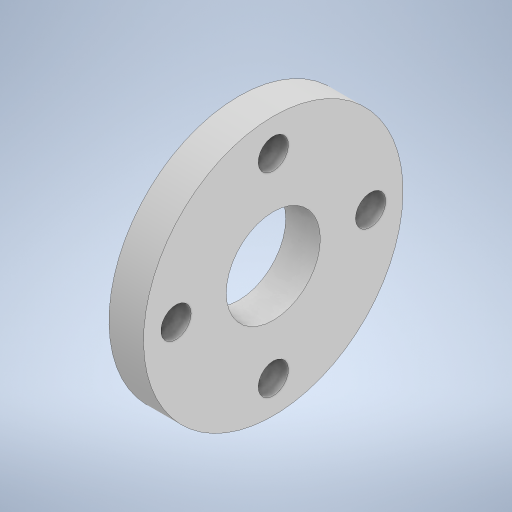
# Autodesk Inventor part: 06-01-2023 flangia piccola
Saved by Autodesk Inventor 2023 (Build 270158000, 158)
## iProperties
Created: 2023-05-31
Part Number: 06-01-2023 flangia piccola
Material: Generico
Document SubType Name: Modeling
Designer: Admin
Density: 1 g/cm^3
Appearance: Default
Author: Admin
Autodesk Inventor part; units mm, degrees
ref_plane "YZ Plane" through (0, 0, 0) normal (1, 0, 0) x (0, 1, 0)
ref_plane "XZ Plane" through (0, 0, 0) normal (0, 1, 0) x (-1, 0, 0)
ref_plane "XY Plane" through (0, 0, 0) normal (0, 0, 1) x (1, 0, 0)
sketch "Schizzo1" plane through (0, 0, 0) normal (0, 0, 1) x (1, 0, 0)
  line L0 (0, 0) -> (22.1221, 0) construction
  line L1 (0, 0) -> (0, 21.75) construction
  line L2 (0, 60) -> (16, 60)
  line L3 (16, 60) -> (16, 21.75)
  line L4 (16, 21.75) -> (0, 21.75)
  line L5 (0, 21.75) -> (0, 60)
  dimension "d0" = 16
  dimension "d1" = 38.25
  dimension "d2" = 120
  constraints: 12 end point, 3 perpendicular, 1 horizontal, 1 parallel, 1 point on line, 1 vertical
  measures "d0" distance of L2.start L2.end
  measures "d1" distance of L2.end L3.end
  measures "d2" diameter of L2 L0
revolve "Rivoluzione1" add sketch "Schizzo1" angle 360 about axis through (0, 0, 0) along (1, 0, 0)
sketch "Schizzo2" plane through (0, 0, 0) normal (1, 0, 0) x (0, 1, 0)
  circle A0 centre (0, 0) radius 45
  circle A1 centre (45, 0) radius 7
  dimension "d4" = 90
  dimension "d5" = 14
  constraints: 2 horizontal alignment, 1 centre point, 1 coincident, 2 other
  measures "d5" diameter of A1
extrude "Estrusione1" cut sketch "Schizzo2" along normal through all contours A0 A1 | A0 A1 picked at (42.7183, -1.3528) picked at (47.059, -1.8371)
pattern_circular "Serie circolare1" count 4 over 360 about axis through (8, 0, 0) along (1, 0, 0) of "Estrusione1"
